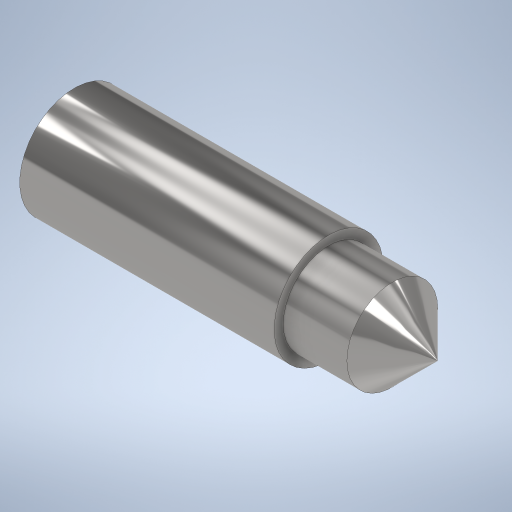
# Autodesk Inventor part: Spitze
Saved by Autodesk Inventor 2024.3 (Build 283343000, 343)
## iProperties
Created: 2025-09-05
Part Number: Spitze
Material: 1.0601 C60
Document SubType Name: Modeling
Designer: Dickert.Jonas
Density: 7.84 g/cm^3
Appearance: Stahl - poliert
Author: Dickert.Jonas
Autodesk Inventor part; units mm, degrees
ref_plane "YZ Plane" through (0, 0, 0) normal (1, 0, 0) x (0, 1, 0)
ref_plane "XZ Plane" through (0, 0, 0) normal (0, 1, 0) x (-1, 0, 0)
ref_plane "XY Plane" through (0, 0, 0) normal (0, 0, 1) x (1, 0, 0)
sketch "Skizze1" plane through (0, 0, 0) normal (0, 0, 1) x (1, 0, 0)
  line L0 (0, 4.0696) -> (0, -0.6783) projected
  line L1 (-4.9592, 0) -> (29.7553, 0) projected
  line L2 (0, 0) -> (0, 3)
  line L3 (0, 3) -> (14, 3)
  line L4 (14, 3) -> (14, 2.5)
  line L5 (14, 2.5) -> (20, 2.5)
  line L6 (20, 2.5) -> (20, 0)
  line L7 (20, 0) -> (16.6087, 3.3913)
  line L8 (20, 0) -> (24.7961, 0) construction
  line L9 (0, 0) -> (20, 0)
  point P0 (17.5, 2.5)
  dimension "d0" = 3
  dimension "d1" = 14
  dimension "d4" = 135
  constraints: 16 end point, 4 perpendicular, 2 point on line, 1 equal length, 1 horizontal
  measures "d0" distance of L2.start L2.end
  measures "d1" distance of L2.end L3.end
  measures "d4" angle of L8 L7
revolve "Umdrehung1" add sketch "Skizze1" angle 360 about axis through (0, 0, 0) along (1, 0, 0) contours L3 L4 L5 L7 L1 L0
